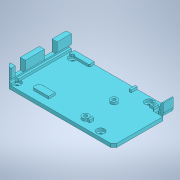
# Autodesk Inventor part: Arduino_holder
Saved by Autodesk Inventor 2022.5 (Build 265521000, 521)
## iProperties
Created: 2023-06-02
Part Number: Arduino_holder
Material: Generic
Document SubType Name: Modeling
Designer: SB13FLLT004
Density: 1 g/cm^3
Appearance: Cadet Blue
Author: SB13FLLT004
Autodesk Inventor part; units mm, degrees
ref_plane "YZ Plane" through (0, 0, 0) normal (1, 0, 0) x (0, 1, 0)
ref_plane "XZ Plane" through (0, 0, 0) normal (0, 1, 0) x (-1, 0, 0)
ref_plane "XY Plane" through (0, 0, 0) normal (0, 0, 1) x (1, 0, 0)
derived "Arduino mega 2560.ipt"
sketch "Sketch: base" plane through (0, 0, 0) normal (0, 1, 0) x (-1, 0, 0)
  line L0 (0, -52.25) -> (0, -1)
  line L1 (-1, 0) -> (-97.96, 0)
  arc A0 (0, -1) -> (-1, 0) centre (-1, -1) ccw
  line L2 (-1, -53.25) -> (-96.26, -53.25)
  arc A1 (-1, -53.25) -> (0, -52.25) centre (-1, -52.25) ccw
  circle A2 centre (-15.4, -50.85) radius 1.6
  circle A3 centre (-14.35, -2.6) radius 1.6
  circle A4 centre (-66.2, -35.65) radius 1.6
  circle A5 centre (-96.4, -2.7) radius 1.6
  circle A6 centre (-90.1, -50.85) radius 1.6
  circle A7 centre (-66.2, -7.7) radius 1.6
  line L3 (-96.26, -53.25) -> (-98.8, -52.4)
  line L4 (-98.8, -52.4) -> (-98.8, -40.65)
  line L5 (-98.8, -40.65) -> (-101.5, -37.8992)
  line L6 (-101.5, -37.8992) -> (-101.5, -5.2492)
  line L7 (-101.5, -5.2492) -> (-98.96, -2.35)
  arc A8 (-97.96, 0) -> (-98.96, -1.08) centre (-97.96, -1.003) ccw
  line L8 (-98.96, -2.35) -> (-98.96, -1.08)
  point P0 (0, 0)
sketch "Sketch: power" plane through (0, 0, 0) normal (0, 1, 0) x (-1, 0, 0)
  line L0 (6.35, -44) -> (-10.05, -44)
  line L1 (-10.05, -44) -> (-10.05, -31.9)
  line L2 (-10.05, -31.9) -> (6.35, -31.9)
  line L3 (6.35, -31.9) -> (6.35, -44)
  line L4 (2.15, -12.65) -> (-12.1, -12.65)
  line L5 (-12.1, -12.65) -> (-12.1, -3.75)
  line L6 (-12.1, -3.75) -> (2.15, -3.75)
  line L7 (2.15, -3.75) -> (2.15, -12.65)
  line L8 (-1, -53.25) -> (-96.26, -53.25)
  line L9 (0, -52.25) -> (0, -1)
  point P0 (0, 0)
sketch "Sketch: pins" plane through (0, 0, 0) normal (0, 1, 0) x (-1, 0, 0)
  line L0 (-26.75, -3.5) -> (-93.25, -3.5)
  line L1 (-93.25, -3.5) -> (-93.25, -1)
  line L2 (-93.25, -1) -> (-26.75, -1)
  line L3 (-26.75, -1) -> (-26.75, -3.5)
  line L4 (-92.75, -52.25) -> (-97.75, -52.25)
  line L5 (-97.75, -52.25) -> (-97.75, -6)
  line L6 (-97.75, -6) -> (-92.75, -6)
  line L7 (-92.75, -6) -> (-92.75, -52.25)
  line L8 (-17.25, -52.25) -> (-87.85, -52.25)
  line L9 (-87.85, -52.25) -> (-87.85, -49.75)
  line L10 (-87.85, -49.75) -> (-17.25, -49.75)
  line L11 (-17.25, -49.75) -> (-17.25, -52.25)
  line L12 (-67.4, -31.25) -> (-62.4, -31.25)
  line L13 (-62.4, -31.25) -> (-62.4, -23.8)
  line L14 (-62.4, -23.8) -> (-67.4, -23.8)
  line L15 (-67.4, -23.8) -> (-67.4, -31.25)
  line L16 (-14.75, -11.3) -> (-3.15, -11.3)
  line L17 (-3.15, -11.3) -> (-3.15, -4.7297)
  line L18 (-5.3879, -1.1) -> (-12.5121, -1.1)
  line L19 (-14.75, -4.7297) -> (-14.75, -11.3)
  line L20 (-16.95, -43.7) -> (-21.95, -43.7)
  line L21 (-21.95, -43.7) -> (-21.95, -48.7)
  line L22 (-21.95, -48.7) -> (-14.5, -48.7)
  line L23 (-14.5, -48.7) -> (-14.5, -43.7)
  line L24 (-1, -53.25) -> (-96.26, -53.25)
  line L25 (-101.5, -37.8992) -> (-101.5, -5.2492)
  line L26 (-1, 0) -> (-97.96, 0)
  line L27 (0, -52.25) -> (0, -1)
  line L28 (-12.5121, -1.1) -> (-12.5121, -4.7297)
  line L29 (-12.5121, -4.7297) -> (-14.75, -4.7297)
  line L30 (-5.3879, -1.1) -> (-5.3879, -4.7297)
  line L31 (-5.3879, -4.7297) -> (-3.15, -4.7297)
  line L32 (-21.95, -43.7) -> (-21.95, -38.7)
  line L33 (-21.95, -38.7) -> (-16.95, -38.7)
  line L34 (-16.95, -38.7) -> (-16.95, -43.7)
  line L35 (-2, -46.75) -> (-9.5, -46.75)
  line L36 (-9.5, -46.75) -> (-9.5, -31.25)
  line L37 (-9.5, -31.25) -> (-2, -31.25)
  line L38 (-2, -31.25) -> (-2, -46.75)
  line L39 (-14.5, -43.7) -> (-16.95, -43.7)
  point P0 (0, 0)
sketch "Sketch: base_" plane through (0, 0, 0) normal (0, 1, 0) x (-1, 0, 0)
  line L0 (2.754, -56.975) -> (1.754, -57.975)
  line L1 (1.754, -57.975) -> (-102.5, -57.975)
  line L2 (2.754, -56.975) -> (2.754, -2.075)
  line L3 (2.754, -2.075) -> (-0.246, 0.925)
  line L4 (-0.246, 0.925) -> (-99.5, 0.925)
  line L5 (-99.5, 0.925) -> (-102.5, -2.075)
  line L6 (-102.5, -2.075) -> (-102.5, -57.975)
  line L7 (-1, -53.25) -> (-96.26, -53.25) construction
  line L8 (-96.26, -53.25) -> (-98.8, -52.4) construction
  line L9 (-98.8, -52.4) -> (-98.8, -40.65) construction
  line L10 (-98.8, -40.65) -> (-101.5, -37.8992) construction
  line L11 (-101.5, -37.8992) -> (-101.5, -5.2492) construction
  arc A0 (-1, -53.25) -> (0, -52.25) centre (-1, -52.25) ccw construction
  line L12 (0, -52.25) -> (0, -1) construction
  arc A1 (0, -1) -> (-1, 0) centre (-1, -1) ccw construction
  line L13 (-1, 0) -> (-97.96, 0) construction
  arc A2 (-97.96, 0) -> (-98.96, -1.08) centre (-97.96, -1.003) ccw construction
  line L14 (-98.96, -2.35) -> (-98.96, -1.08) construction
  line L15 (-101.5, -5.2492) -> (-98.96, -2.35) construction
  circle A3 centre (-14.35, -2.6) radius 1.65
  circle A4 centre (-15.4, -50.85) radius 1.65
  circle A5 centre (-66.2, -35.65) radius 1.65
  circle A6 centre (-66.2, -7.7) radius 1.65
  circle A7 centre (-96.4, -2.7) radius 1.65
  circle A8 centre (-90.1, -50.85) radius 1.65
  line L16 (-102.5, -47.175) -> (-92.8, -47.175)
  line L17 (-92.8, -47.175) -> (-92.8, -47.975)
  line L18 (-92.8, -47.975) -> (-102.5, -47.975)
  point P0 (0, 0)
  point P1 (-14.35, -2.6)
  dimension "d2" = 135
  dimension "d5" = 1
  dimension "d7" = 135
  dimension "d9" = 3
  dimension "d10" = 135
  dimension "d11" = 3
  dimension "d13" = 105.254
  dimension "d18" = 58.9
  dimension "d19" = 1
  dimension "d22" = 0.925
  dimension "d100" = 3.3
  dimension "d131" = 7.125
  dimension "d184" = 0.8
  dimension "d185" = 10
  dimension "d186" = 9.7
  constraints: 20 end point, 6 centre point, 6 coincident, 6 perpendicular, 5 equal radius, 2 point on line, 1 horizontal
  measures "d2" angle of L1 L0
  measures "d5" horizontal distance of L0.start L0.end
  measures "d7" angle of L5 L6
  measures "d9" horizontal distance of L4.end L5.end
  measures "d10" angle of L4 L3
  measures "d11" horizontal distance of L2.end L3.end
  measures "d13" distance between parallel lines of L2 L6
  measures "d18" distance between parallel lines of L4 L1
  measures "d19" distance between parallel lines of L6 L11
  measures "d22" distance between parallel lines of L4 L13
  measures "d100" diameter of A3
  measures "d131" distance from line of L1 point (-15.4, -50.85)
  measures "d184" distance of L16.end L17.end
  measures "d185" distance between parallel lines of L18 L1
  measures "d186" distance of L17.end L18.end
sketch "Sketch: front wall" plane through (0, 0, 0) normal (0, 1, 0) x (-1, 0, 0)
  line L0 (0, 0.925) -> (0, -57.975)
  line L1 (0, -57.975) -> (2, -57.975)
  line L2 (2, -57.975) -> (3, -56.975)
  line L3 (3, -56.975) -> (3, -2.075)
  line L4 (3, -2.075) -> (0, 0.925)
  line L5 (0, 0.925) -> (0, 0.925)
  circle A0 centre (-14.35, -2.6) radius 1.65 construction
  line L6 (-0.246, 0.925) -> (-99.5, 0.925) construction
  line L7 (1.754, -57.975) -> (-102.5, -57.975) construction
  line L8 (0, 0.925) -> (-2, 0.925)
  line L9 (-2, 0.925) -> (-2, -57.975)
  line L10 (-2, -57.975) -> (0, -57.975)
  point P0 (0, 0)
  dimension "d140" = 14.35
  dimension "d141" = 135
  dimension "d142" = 135
  dimension "d143" = 1
  dimension "d144" = 3
  dimension "d152" = 2
  dimension "d153" = 5
  constraints: 18 end point, 6 perpendicular, 2 collinear, 1 vertical
  measures "d140" distance from line of L0 A0.centre
  measures "d141" angle of L4 L5
  measures "d142" angle of L1 L2
  measures "d143" horizontal distance of L1.end L2.end
  measures "d144" horizontal distance of L3.end L4.end
  measures "d152" distance between parallel lines of L9 L0
  measures "d153" distance between parallel lines of L3 L9
sketch "Sketch: front power wall" plane through (0, 0, 0) normal (1, 0, 0) x (0, 1, 0)
  line L0 (0, 0.925) -> (18.4, 0.925)
  line L1 (18.4, 0.925) -> (18.4, -3.356)
  line L2 (18.4, -3.356) -> (7.55, -3.356)
  line L3 (7.55, -3.356) -> (7.55, -12.856)
  line L4 (7.55, -12.856) -> (18.4, -12.856)
  line L5 (18.4, -12.856) -> (18.4, -31.606)
  line L6 (18.4, -31.606) -> (7.55, -31.606)
  line L7 (7.55, -31.606) -> (7.55, -44.106)
  line L8 (7.55, -44.106) -> (18.4, -44.106)
  line L9 (18.4, -44.106) -> (18.4, -57.975)
  line L10 (18.4, -57.975) -> (0, -57.975)
  line L11 (0, -57.975) -> (0, 0.925)
  line L12 (18.4, -3.356) -> (18.4, -12.856)
  line L13 (18.4, -31.606) -> (18.4, -44.106)
  point P0 (0, 0)
  point P1 (0, -2.6)
  dimension "d51" = 9.5
  dimension "d88" = 12.5
  dimension "d89" = 18.4
  dimension "d154" = 7.55
  dimension "d155" = 0.756
  dimension "d156" = 18.75
  constraints: 28 end point, 8 perpendicular, 3 collinear, 2 coincident, 1 horizontal, 1 vertical
  measures "d51" distance of L2.end L3.end
  measures "d88" distance of L6.end L7.end
  measures "d89" distance of L0.start L0.end
  measures "d154" distance between parallel lines of L11 L3
  measures "d155" distance from line of L2 point (0, -2.6)
  measures "d156" distance between parallel lines of L6 L4
sketch "Sketch: hole popup" plane through (0, 0, 0) normal (0, 1, 0) x (-1, 0, 0)
  circle A0 centre (-15.4, -50.85) radius 1.6 construction
  circle A1 centre (-14.35, -2.6) radius 1.6 construction
  circle A2 centre (-66.2, -7.7) radius 1.6 construction
  circle A3 centre (-66.2, -35.65) radius 1.6 construction
  circle A4 centre (-96.4, -2.7) radius 1.6 construction
  line L0 (-87.85, -49.75) -> (-17.25, -49.75) construction
  line L1 (-87.85, -52.25) -> (-87.85, -49.75) construction
  line L2 (-17.25, -52.25) -> (-87.85, -52.25) construction
  line L3 (-17.25, -49.75) -> (-17.25, -52.25) construction
  line L4 (-92.75, -6) -> (-92.75, -52.25) construction
  line L5 (-97.75, -52.25) -> (-97.75, -6) construction
  line L6 (-97.75, -6) -> (-92.75, -6) construction
  line L7 (-92.75, -52.25) -> (-97.75, -52.25) construction
  line L8 (-26.75, -3.5) -> (-93.25, -3.5) construction
  line L9 (-93.25, -1) -> (-26.75, -1) construction
  line L10 (-93.25, -3.5) -> (-93.25, -1) construction
  line L11 (-26.75, -1) -> (-26.75, -3.5) construction
  line L12 (-16.95, -38.7) -> (-16.95, -43.7) construction
  line L13 (-21.95, -38.7) -> (-16.95, -38.7) construction
  line L14 (-21.95, -43.7) -> (-21.95, -38.7) construction
  line L15 (-21.95, -43.7) -> (-21.95, -48.7) construction
  line L16 (-21.95, -48.7) -> (-14.5, -48.7) construction
  line L17 (-14.5, -48.7) -> (-14.5, -43.7) construction
  line L18 (-14.5, -43.7) -> (-21.95, -43.7) construction
  line L19 (-9.5, -46.75) -> (-9.5, -31.25) construction
  line L20 (-2, -46.75) -> (-9.5, -46.75) construction
  line L21 (-2, -31.25) -> (-2, -46.75) construction
  line L22 (-9.5, -31.25) -> (-2, -31.25) construction
  line L23 (-5.3879, -4.7297) -> (-3.15, -4.7297) construction
  line L24 (-5.3879, -1.1) -> (-5.3879, -4.7297) construction
  line L25 (-12.5121, -1.1) -> (-12.5121, -4.7297) construction
  line L26 (-12.5121, -4.7297) -> (-14.75, -4.7297) construction
  line L27 (-14.75, -11.3) -> (-3.15, -11.3) construction
  line L28 (-5.3879, -1.1) -> (-12.5121, -1.1) construction
  line L29 (-14.75, -4.7297) -> (-14.75, -11.3) construction
  line L30 (-3.15, -11.3) -> (-3.15, -4.7297) construction
  line L31 (-14.5, -43.7) -> (-16.95, -43.7) construction
  line L32 (-67.4, -31.25) -> (-62.4, -31.25) construction
  line L33 (-67.4, -23.8) -> (-67.4, -31.25) construction
  line L34 (-62.4, -31.25) -> (-62.4, -23.8) construction
  line L35 (-62.4, -23.8) -> (-67.4, -23.8) construction
  line L36 (-88, -53.05) -> (-92.4, -53.05)
  line L37 (-92.4, -53.05) -> (-92.4, -48.65)
  line L38 (-92.4, -48.65) -> (-88, -48.65)
  line L39 (-88, -48.65) -> (-88, -53.05)
  circle A5 centre (-90.2, -50.85) radius 1.15
  circle A6 centre (-90.1, -50.85) radius 1.6 construction
  point P0 (0, 0)
  point P1 (-90.2, -53.05)
  point P2 (-88, -50.85)
  dimension "d94" = 4.4
  dimension "d95" = 2.3
  dimension "d157" = 2.2
  dimension "d158" = 2.2
  dimension "d159" = 4.4
  dimension "d181" = 0.1
  constraints: 8 end point, 3 equal length, 2 horizontal alignment, 2 midpoint, 1 centre point, 1 horizontal, 1 perpendicular, 1 vertical alignment
  measures "d94" distance of L38.end L36.start
  measures "d95" diameter of A5
  measures "d157" distance from line of L39 point (-90.2, -53.05)
  measures "d158" distance of L36.end point (-90.2, -53.05)
  measures "d159" distance of L36.start L36.end
  measures "d181" distance of A6.centre A5.centre
sketch "Sketch: prop up" plane through (0, 0, 0) normal (0, 1, 0) x (-1, 0, 0)
  line L0 (-64.72, -57.975) -> (-66.72, -57.975)
  line L1 (-66.72, -57.975) -> (-66.72, -51.975)
  line L2 (-66.72, -51.975) -> (-64.72, -51.975)
  line L3 (-64.72, -51.975) -> (-64.72, -57.975)
  line L4 (-70, -10.125) -> (-72, -10.125)
  line L5 (-72, -10.125) -> (-72, -6.125)
  line L6 (-72, -6.125) -> (-70, -6.125)
  line L7 (-70, -6.125) -> (-70, -10.125)
  line L8 (-16.745, -6.125) -> (-31.495, -6.125)
  line L9 (-31.495, -6.125) -> (-31.495, -12.575)
  line L10 (-31.495, -12.575) -> (-19.745, -12.575)
  line L11 (-15.745, -8.575) -> (-15.745, -7.125)
  line L12 (-15.745, -7.125) -> (-16.745, -6.125)
  line L13 (-0.246, 0.925) -> (-99.5, 0.925) construction
  arc A0 (-19.745, -12.575) -> (-15.745, -8.575) centre (-19.745, -8.575) ccw
  circle A1 centre (-14.35, -2.6) radius 1.65 construction
  circle A2 centre (-19.745, -8.575) radius 1.6
  line L14 (-102.5, -2.075) -> (-102.5, -57.975) construction
  line L15 (1.754, -57.975) -> (-102.5, -57.975) construction
  line L16 (-92.935, -6.125) -> (-102.5, -6.125)
  line L17 (-102.5, -6.125) -> (-102.5, -12.575)
  line L18 (-102.5, -12.575) -> (-96.185, -12.575)
  arc A3 (-96.185, -12.575) -> (-92.935, -9.325) centre (-96.185, -9.325) ccw
  line L19 (-92.935, -9.325) -> (-92.935, -6.125)
  line L20 (-5.2356, -57.975) -> (-24.4856, -57.975)
  line L21 (-24.4856, -57.975) -> (-24.4856, -53.975)
  line L22 (-24.4856, -53.975) -> (-23.4856, -52.975)
  line L23 (-23.4856, -52.975) -> (-5.2356, -52.975)
  line L24 (-5.2356, -52.975) -> (-5.2356, -57.975)
  circle A4 centre (-66.2, -7.7) radius 3.25
  circle A5 centre (-66.2, -35.65) radius 3.25
  circle A6 centre (-66.2, -7.7) radius 1.65 projected
  circle A7 centre (-66.2, -35.65) radius 1.65 projected
  point P0 (0, 0)
  point P1 (-15.4, -50.85)
  point P2 (-96.4, -2.7)
  dimension "d101" = 6.45
  dimension "d103" = 1
  dimension "d104" = 135
  dimension "d105" = 14.75
  dimension "d106" = 5.395
  dimension "d107" = 5.975
  dimension "d108" = 3.2
  dimension "d110" = 2
  dimension "d111" = 4
  dimension "d115" = 2
  dimension "d116" = 6
  dimension "d118" = 6.45
  dimension "d119" = 3.25
  dimension "d121" = 9.565
  dimension "d127" = 135
  dimension "d128" = 4
  dimension "d129" = 19.25
  dimension "d130" = 1
  dimension "d132" = 9.0856
  dimension "d134" = 0.52
  dimension "d135" = 3.8
  dimension "d136" = 2.425
  dimension "d138" = 3.425
  dimension "d139" = 3.525
  dimension "d160" = 6.5
  constraints: 44 end point, 15 perpendicular, 5 centre point, 5 horizontal, 4 point on circle, 4 tangent, 3 coincident, 3 collinear, 1 equal radius
  measures "d101" distance of L8.end L9.end
  measures "d103" horizontal distance of L11.end L8.start
  measures "d104" angle of L8 L12
  measures "d105" distance of L8.start L8.end
  measures "d106" horizontal distance of A2.centre A1.centre
  measures "d107" vertical distance of A1.centre A2.centre
  measures "d108" diameter of A2
  measures "d110" distance of L5.end L6.end
  measures "d111" distance of L6.end L4.start
  measures "d115" distance of L0.start L0.end
  measures "d116" distance of L0.end L1.end
  measures "d118" distance between parallel lines of L16 L18
  measures "d119" radius of A3
  measures "d121" distance of L16.start L16.end
  measures "d127" angle of L22 L21
  measures "d128" distance of L20.end L21.end
  measures "d129" distance of L20.start L20.end
  measures "d130" horizontal distance of L21.end L22.end
  measures "d132" distance from line of L21 point (-15.4, -50.85)
  measures "d134" distance from line of point (-66.2, -35.65) L1
  measures "d135" distance from line of point (-66.2, -7.7) L7
  measures "d136" distance from line of point (-66.2, -7.7) L4
  measures "d138" distance from line of L16 point (-96.4, -2.7)
  measures "d139" distance from line of A1.centre L8
  measures "d160" diameter of A4
sketch "Sketch: front wall cutout" plane through (0, 0, 0) normal (0, 0, 1) x (1, 0, 0)
  line L0 (5.2582, 12.6082) -> (-0.05, 7.3)
  line L1 (-0.05, 7.3) -> (-0.05, 5.9)
  line L2 (-0.05, 5.9) -> (5.2582, 5.9)
  line L3 (5.2582, 5.9) -> (5.2582, 12.6082)
  point P0 (0, 0)
  point P1 (14.35, 0)
  dimension "d122" = 135
  dimension "d124" = 1.4
  dimension "d150" = 5.9
  dimension "d151" = 14.4
  constraints: 8 end point, 2 perpendicular, 1 vertical
  measures "d122" angle of L1 L0
  measures "d124" distance of L0.end L1.end
  measures "d150" distance from line of L2 point (0, 0)
  measures "d151" distance from line of L1 point (14.35, 0)
extrude "Ex: base" add sketch "Sketch: base_" along normal blind 3.5 contours L0 L1 L6 L18 L17 L16 L5 L4 L3 L2 | A3 | A4 | A5 | A6 | A7 | A8
extrude "Ex: front wall build" add sketch "Sketch: front wall" along normal blind 18.4
extrude "Ex: front wall cut" cut sketch "Sketch: front power wall" along normal through all both and the other way through all contours L12 L4 L3 L2 | L8 L7 L6 L13
extrude "Ex: hole popup1" add sketch "Sketch: hole popup" along normal blind 5.9 contours L36 L37 L38 L39 | A5
extrude "Ex: hole popup2" add sketch "Sketch: hole popup" along normal blind 8.4 contours A5
extrude "Ex: prop up" add sketch "Sketch: prop up" along normal blind 5.9 contours L0 L1 L2 L3 | L4 L5 L6 L7 | L12 L11 A0 L10 L9 L8 | A2 | L20 L21 L22 L23 L24 | A4 | A5
extrude "Ex: front wall cutout" cut sketch "Sketch: front wall cutout" along normal through all both and the other way through all
sketch "Sketch: ramp" plane through (0, 0, 0) normal (0, 0, 1) x (1, 0, 0)
  line L0 (99.7338, 13) -> (101.0551, 14.5)
  line L1 (101.0551, 14.5) -> (102.0551, 14.5)
  line L2 (102.0551, 14.5) -> (102.0551, 5.9)
  arc A0 (96.55, 1.8947) -> (99.6551, 5.9) centre (94.3907, 6.775) ccw
  line L3 (98.2, 7.65) -> (99.6551, 7.65)
  line L4 (99.6551, 7.65) -> (99.6551, 5.9)
  line L5 (99.7338, 13) -> (96.55, 1.8947)
  line L6 (96.55, 1.8947) -> (93.9053, 1.8947)
  line L7 (93.9053, 1.8947) -> (92.4, 3.4)
  line L8 (92.4, 3.4) -> (92.4, 5.9)
  line L9 (97, 2.1197) -> (98.5855, 7.65)
  line L10 (92.4, 3.5) -> (92.4, 5.9) projected
  line L11 (92.4, 6.697) -> (92.4, 0)
  line L12 (102.5, 3.5) -> (66.72, 3.5) projected
  line L13 (102.5, 0) -> (102.5, 3.5) projected
  line L14 (102.5, 0) -> (-2, 0) projected
  arc A1 (96.1551, 0) -> (102.0551, 5.9) centre (96.1551, 5.9) ccw
  point P0 (0, 0)
  point P1 (92.4, 3.4)
  point P2 (97.0102, 3.5)
  point P3 (98.6043, 3.5)
  point P4 (97.3957, 3.5)
  point P5 (96.4, 0)
  point P6 (92.4, 3.5)
  point P7 (101.5449, 3.5)
  dimension "d161" = 1
  dimension "d162" = 135
  dimension "d163" = 105.997
  dimension "d164" = 8.6
  dimension "d165" = 6.85
  dimension "d166" = 1.5
  dimension "d168" = 2.5
  dimension "d169" = 1.5053
  dimension "d170" = 2.6447
  dimension "d171" = 1.75
  dimension "d172" = 0.45
  dimension "d173" = 4.0053
  dimension "d175" = 2.4
  dimension "d180" = 1.4551
  dimension "d183" = 0.15
  dimension "d195" = 0.4449
  dimension "d196" = 4.3
  dimension "d197" = 4.15
  constraints: 22 end point, 6 point on circle, 4 point on line, 3 horizontal, 3 vertical, 2 centre point, 2 tangent, 1 collinear, 1 parallel, 1 perpendicular
  measures "d161" distance of L0.end L1.end
  measures "d162" angle of L6 L7
  measures "d163" angle of L6 L5
  measures "d164" distance of L1.end L2.end
  measures "d165" distance between parallel lines of L1 L3
  measures "d166" vertical distance of L0.start L0.end
  measures "d168" distance of L8.end L7.end
  measures "d169" horizontal distance of L6.end L7.end
  measures "d170" distance of L5.end L6.end
  measures "d171" distance of L3.end L4.end
  measures "d172" horizontal distance of L5.end L9.start
  measures "d173" vertical distance of L4.end L5.end
  measures "d175" distance between parallel lines of L2 L4
  measures "d180" distance of L3.start L3.end
  measures "d183" horizontal distance of L5.end point (96.4, 0)
  measures "d195" distance between parallel lines of L2 L13
  measures "d196" distance from line of L13 L3.start
  measures "d197" distance between parallel lines of L12 L3
extrude "Ex: ramp" add sketch "Sketch: ramp" along normal blind 10 from surface at -57.975 contours L0 L1 L2 A1 L12 A0 L4 L3 L5 | L3 L9 L12 L5
extrude "Ex: ramp cutout" cut sketch "Sketch: ramp" along normal blind 10 from surface at -57.975 contours L5 L6 L7 L8 L12 | L12 L13 L14 A1
sketch "Sketch: mounting to PCB Arduino" plane through (0, 3.5, 0) normal (0, -1, 0) x (1, 0, 0)
  circle A0 centre (84.15, -4.55) radius 1.6 projected
  circle A1 centre (83.1, -52.8) radius 1.6 projected
  circle A2 centre (8.4, -52.8) radius 1.6 projected
  circle A3 centre (2.1, -4.65) radius 1.6 projected
  circle A4 centre (84.15, -4.55) radius 1.65
  circle A5 centre (83.1, -52.8) radius 1.65
  circle A6 centre (8.4, -52.8) radius 1.65
  circle A7 centre (2.1, -4.65) radius 1.65
  circle A8 centre (8.4, -52.8) radius 3.81
  circle A9 centre (83.1, -52.8) radius 3.81
  circle A10 centre (2.1, -4.65) radius 3.81
  circle A11 centre (84.15, -4.55) radius 3.81
  point P0 (0, 0)
  dimension "d187" = 3.3
  dimension "d190" = 7.62
  constraints: 8 centre point, 8 coincident, 6 equal radius
  measures "d187" diameter of A7
  measures "d190" diameter of A11
extrude "Ex: countersink for standoffs" cut sketch "Sketch: mounting to PCB Arduino" along normal blind 2.75 contours A8 | A9 | A10 | A11
sketch "Sketch15" plane through (0, 0, 0) normal (0, -1, 0) x (1, 0, 0)
  circle A0 centre (2.1, -4.65) radius 1.65 projected
  circle A1 centre (8.4, -52.8) radius 1.65 projected
  circle A2 centre (83.1, -52.8) radius 1.65 projected
  circle A3 centre (84.15, -4.55) radius 1.65 projected
  point P0 (0, 0)
extrude "Ex: holes for mounting" cut sketch "Sketch15" along normal through all both and the other way through all
sketch "Sketch3" plane through (0, 0, 0) normal (1, 0, 0) x (0, 1, 0)
  circle A0 centre (8.1, -8.2) radius 4.45 projected
  line L0 (0, -12.65) -> (0, -3.75) projected
  line L1 (17.2286, -3.75) -> (0, -3.75) projected
  line L2 (17.2286, -12.65) -> (0, -12.65) projected
  line L3 (17.2286, -3.75) -> (17.2286, -12.65) projected
  line L4 (12.55, -3.117) -> (12.55, -13.9417) construction
  point P0 (0, 0)
  point P1 (0, -8.2)
body "Solid1"
